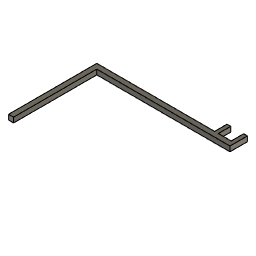
basic stress test bracket non-triangular v2 (Autodesk Fusion 360 design; units mm, degrees)
Autodesk Fusion 360 part; units mm, degrees
note: some values were not read from the file. Set by a fixed rule: which sketch regions a step uses.
sketch "Sketch1" plane through (0, 0, 0) normal (0, 0, 1) x (1, 0, 0)
  line L0 (0, 0) -> (7.62, 0)
  line L1 (7.62, 0) -> (7.62, 134.62)
  line L2 (7.62, 134.62) -> (0, 134.62)
  line L3 (0, 134.62) -> (0, 0)
  line L4 (7.62, 134.62) -> (210.82, 134.62)
  line L5 (210.82, 134.62) -> (210.82, 127)
  line L6 (210.82, 127) -> (7.62, 127)
  line L7 (7.62, 127) -> (7.62, 134.62)
  line L8 (7.62, 0) -> (3.5814, 6.4617)
  line L9 (206.7814, 133.4617) -> (210.82, 127)
  line L10 (210.82, 134.62) -> (205.105, 134.62)
  line L11 (205.105, 134.62) -> (205.105, 153.67)
  line L12 (205.105, 153.67) -> (210.82, 153.67)
  line L13 (210.82, 153.67) -> (210.82, 134.62)
  line L14 (185.42, 134.62) -> (179.705, 134.62)
  line L15 (179.705, 134.62) -> (179.705, 153.6683)
  line L16 (179.705, 153.6683) -> (185.42, 153.6683)
  line L17 (185.42, 153.6683) -> (185.42, 134.62)
  dimension "d1" = 134.62
  dimension "d2" = 7.62
  dimension "d3" = 203.2
  dimension "d4" = 7.62
  dimension "d5" = 5.715
  dimension "d6" = 19.05
  dimension "d7" = 19.0483
  dimension "d8" = 5.715
  constraint horizontal L0
  constraint vertical L1
  constraint horizontal L2
  constraint vertical L3
  constraint coincident L0.start L3.end
  constraint horizontal L4
  constraint vertical L5
  constraint horizontal L6
  constraint vertical L7
  constraint parallel L8 L9
  constraint horizontal L10
  constraint vertical L11
  constraint horizontal L12
  constraint vertical L13
  constraint horizontal L14
  constraint vertical L15
  constraint horizontal L16
  constraint vertical L17
  measures "d1" distance of L0.start L2.end
  measures "d2" distance of L0.start L0.end
  measures "d3" distance of L1.end L4.end
  measures "d4" distance of L5.end L9.start
  measures "d5" distance of L4.end L10.end
  measures "d6" distance of L4.end L12.end
  measures "d7" distance of L14.start L16.end
  measures "d8" distance of L14.start L14.end
extrude "Extrude1" add sketch "Sketch1" along normal blind 7.62
